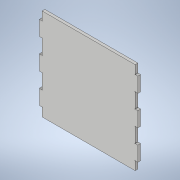
# Autodesk Inventor part: bottom-case
Saved by Autodesk Inventor 2020 (Build 240168000, 168)
## iProperties
Created: 2019-12-17
Part Number: bottom-case
Material: Generic
Document SubType Name: Modeling
Designer: fabfarm
Density: 1 g/cm^3
Appearance: Default
Author: fabfarm
Autodesk Inventor part; units mm, degrees
ref_plane "YZ Plane" through (0, 0, 0) normal (1, 0, 0) x (0, 1, 0)
ref_plane "XZ Plane" through (0, 0, 0) normal (0, 1, 0) x (-1, 0, 0)
ref_plane "XY Plane" through (0, 0, 0) normal (0, 0, 1) x (1, 0, 0)
sketch "Sketch1" plane through (0, 0, 0) normal (0, 0, 1) x (1, 0, 0)
  line L0 (330, -307.45) -> (-330, -307.45)
  line L1 (-330, -307.45) -> (-330, 307.45)
  line L2 (-330, 307.45) -> (330, 307.45)
  line L3 (330, 307.45) -> (330, -307.45)
  line L4 (330, -307.45) -> (-330, 307.45) construction
  line L5 (-330, -307.45) -> (330, 307.45) construction
  point P0 (0, 0)
  dimension "d0" = 614.9
  dimension "d1" = 660
  constraints: 12 end point, 2 midpoint, 2 parallel, 1 horizontal, 1 perpendicular
  measures "d0" distance of L2.end L0.start
  measures "d1" distance of L0.start L0.end
extrude "Extrusion1" add sketch "Sketch1" along normal blind 18.55
sketch "Sketch2" plane through (0, 0, 18.55) normal (0, 0, 1) x (1, 0, 0)
  line L0 (-330, 307.45) -> (-330, -307.45) construction
  line L1 (330, 307.45) -> (-330, 307.45) construction
  line L2 (-330, 307.45) -> (-311.45, 307.45)
  line L3 (-311.45, 307.45) -> (-311.45, 250)
  line L4 (-311.45, 250) -> (-330, 250)
  line L5 (-330, 250) -> (-330, 307.45)
  line L6 (-330, -307.45) -> (330, -307.45) projected
  line L7 (-330, -307.45) -> (-311.45, -307.45)
  line L8 (-311.45, -307.45) -> (-311.45, -250)
  line L9 (-311.45, -250) -> (-330, -250)
  line L10 (-330, -250) -> (-330, -307.45)
  line L11 (-330, -150) -> (-311.45, -150)
  line L12 (-311.45, -150) -> (-311.45, -50)
  line L13 (-311.45, -50) -> (-330, -50)
  line L14 (-330, -50) -> (-330, -150)
  line L15 (-330, 50) -> (-311.45, 50)
  line L16 (-311.45, 50) -> (-311.45, 150)
  line L17 (-311.45, 150) -> (-330, 150)
  line L18 (-330, 150) -> (-330, 50)
  point P0 (0, 0)
  dimension "d21" = 100
  dimension "d22" = 100
  dimension "d23" = 100
  dimension "d24" = 100
  dimension "d25" = 57.45
  dimension "d26" = 18.55
  constraints: 32 end point, 8 parallel, 5 point on line, 4 horizontal, 4 perpendicular, 3 collinear
  measures "d21" distance between parallel lines of L4 L17
  measures "d22" distance of L15.end L16.end
  measures "d23" distance between parallel lines of L13 L15
  measures "d24" distance of L11.end L12.end
  measures "d25" distance of L2.end L3.end
  measures "d26" distance of L0.end L7.end
extrude "Extrusion2" cut sketch "Sketch2" against normal blind 18.55
mirror "Mirror1" about plane through (0, 0, 0) normal (1, 0, 0) of "Extrusion2"
sketch "Sketch3" plane through (0, 0, 18.55) normal (0, 0, 1) x (1, 0, 0)
  line L0 (-330, -307.45) -> (-330, 307.45) projected
  line L1 (-330, 305) -> (-311.45, 305) projected
  line L2 (-330, 307.45) -> (-311.45, 307.45)
  line L3 (-311.45, 307.45) -> (-311.45, 305)
  line L4 (-311.45, 305) -> (-330, 305)
  line L5 (-330, 305) -> (-330, 307.45)
  line L6 (311.45, 305) -> (330, 305) projected
  line L7 (-330, 307.45) -> (330, 307.45) projected
  line L8 (311.45, 305) -> (330, 305)
  line L9 (330, 305) -> (330, 307.45)
  line L10 (330, 307.45) -> (311.45, 307.45)
  line L11 (311.45, 307.45) -> (311.45, 305)
  point P0 (0, 0)
  constraints: 16 end point, 4 parallel, 2 horizontal, 2 perpendicular
extrude "Extrusion3" cut sketch "Sketch3" against normal blind 50
sketch "Sketch4" plane through (0, 0, 18.55) normal (0, 0, 1) x (1, 0, 0)
  line L0 (-330, -307.45) -> (330, -307.45) projected
  line L1 (-330, -307.45) -> (-311.45, -307.45)
  line L2 (-311.45, -307.45) -> (-311.45, -255)
  line L3 (-311.45, -255) -> (-330, -255)
  line L4 (-330, -255) -> (-330, -307.45)
  line L5 (-311.45, -215) -> (-311.45, -235) projected
  line L6 (-311.45, -235) -> (-330, -235) projected
  line L7 (330, -307.45) -> (311.45, -307.45)
  line L8 (311.45, -307.45) -> (311.45, -255)
  line L9 (311.45, -255) -> (330, -255)
  line L10 (330, -255) -> (330, -307.45)
  line L11 (311.45, -235) -> (311.45, -215) projected
  point P0 (0, 0)
  dimension "d18" = 20
  constraints: 16 end point, 4 parallel, 3 collinear, 2 horizontal, 2 perpendicular
  measures "d18" distance between parallel lines of L3 L6
extrude "Extrusion4" cut sketch "Sketch4" against normal blind 50
sketch "Esquisse5" plane through (0, 0, 18.55) normal (0, 0, 1) x (1, 0, 0)
  line L0 (-330, 250) -> (-311.45, 250) projected
  circle A0 centre (-311.45, 250) radius 1.59
  line L1 (-311.45, 150) -> (-330, 150) projected
  circle A1 centre (-311.45, 150) radius 1.59
  line L2 (-330, 50) -> (-311.45, 50) projected
  circle A2 centre (-311.45, 50) radius 1.59
  line L3 (-311.45, -50) -> (-330, -50) projected
  circle A3 centre (-311.45, -50) radius 1.59
  line L4 (-311.45, -150) -> (-311.45, -50) projected
  circle A4 centre (-311.45, -150) radius 1.59
  line L5 (-311.45, -307.45) -> (-311.45, -250) projected
  circle A5 centre (-311.45, -250) radius 1.59
  line L6 (-311.45, 307.45) -> (311.45, 307.45) projected
  line L7 (0, 307.45) -> (0, -307.45) construction
  line L8 (311.45, -307.45) -> (-311.45, -307.45) projected
  line L9 (330, 250) -> (311.45, 250)
  circle A6 centre (311.45, 250) radius 1.59
  line L10 (311.45, 150) -> (330, 150)
  circle A7 centre (311.45, 150) radius 1.59
  line L11 (330, 50) -> (311.45, 50)
  circle A8 centre (311.45, 50) radius 1.59
  line L12 (311.45, -50) -> (330, -50)
  circle A9 centre (311.45, -50) radius 1.59
  line L13 (311.45, -150) -> (311.45, -50)
  circle A10 centre (311.45, -150) radius 1.59
  line L14 (311.45, -307.45) -> (311.45, -250)
  circle A11 centre (311.45, -250) radius 1.59
  point P0 (0, 0)
  dimension "d27" = 3.18
  constraints: 14 end point, 12 centre point, 10 symmetric about line, 5 equal radius, 2 midpoint, 6 other
  measures "d27" diameter of A0
extrude "Extrusion5" cut sketch "Esquisse5" against normal blind 18.55
body "Solid1"
